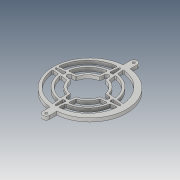
# Autodesk Inventor part: verticalThrusterCover2
Saved by Autodesk Inventor 2018 (Build 220112000, 112)
## iProperties
Created: 2020-02-09
Part Number: verticalThrusterCover2
Material: Generic
Document SubType Name: Modeling
Designer: anirudh
Density: 1 g/cm^3
Appearance: Default
Author: anirudh
Autodesk Inventor part; units mm, degrees
ref_plane "YZ Plane" through (0, 0, 0) normal (1, 0, 0) x (0, 1, 0)
ref_plane "XZ Plane" through (0, 0, 0) normal (0, 1, 0) x (-1, 0, 0)
ref_plane "XY Plane" through (0, 0, 0) normal (0, 0, 1) x (1, 0, 0)
sketch "Sketch1" plane through (0, 0, 0) normal (0, 1, 0) x (-1, 0, 0)
  circle A0 centre (0, -63.5) radius 1.75
  circle A1 centre (0, 63.5) radius 1.75
  circle A2 centre (0, -63.5) radius 1.75
  circle A3 centre (0, 63.5) radius 1.75
  arc A4 (5.08, 63.5) -> (-5.08, 63.5) centre (0, 63.5) ccw
  arc A5 (-5.08, -63.5) -> (5.08, -63.5) centre (0, -63.5) ccw
  line L0 (5.08, 63.5) -> (5.08, 53.0975)
  line L1 (5.08, -53.0975) -> (5.08, -63.5)
  line L2 (-5.08, -63.5) -> (-5.08, -53.0975)
  line L3 (-5.08, 53.0975) -> (-5.08, 63.5)
  arc A6 (-5.08, 53.0975) -> (-5.08, -53.0975) centre (0, 0) ccw
  arc A7 (5.08, -53.0975) -> (5.08, 53.0975) centre (0, 0) ccw
  arc A8 (-0.1848, -27.646) -> (6.1284, -27.646) centre (2.9718, -27.305) ccw
  line L4 (6.8199, -21.2443) -> (6.1284, -27.646)
  line L5 (-0.1848, -27.646) -> (-0.8763, -21.2443)
  line L6 (30.6178, -3.1566) -> (24.2161, -3.8481)
  line L7 (24.2161, 3.8481) -> (30.6178, 3.1566)
  arc A9 (30.6178, -3.1566) -> (30.6178, 3.1566) centre (30.2768, 0) ccw
  line L8 (6.1284, 27.646) -> (6.8199, 21.2443)
  line L9 (-0.8763, 21.2443) -> (-0.1848, 27.646)
  arc A10 (6.1284, 27.646) -> (-0.1848, 27.646) centre (2.9718, 27.305) ccw
  line L10 (-24.6742, 3.1566) -> (-18.2725, 3.8481)
  line L11 (-18.2725, -3.8481) -> (-24.6742, -3.1566)
  arc A11 (-24.6742, 3.1566) -> (-24.6742, -3.1566) centre (-24.3332, 0) ccw
  arc A12 (24.2161, 3.8481) -> (6.8199, 21.2443) centre (2.9718, 0) ccw
  arc A13 (-0.8763, 21.2443) -> (-18.2725, 3.8481) centre (2.9718, 0) ccw
  arc A14 (-18.2725, -3.8481) -> (-0.8763, -21.2443) centre (2.9718, 0) ccw
  arc A15 (6.8199, -21.2443) -> (24.2161, -3.8481) centre (2.9718, 0) ccw
  dimension "d34" = 360
  constraints: 24 end point, 24 point on circle, 16 centre point, 4 coincident, 4 vertical, 2 concentric, 33 other
extrude "Extrusion2" add sketch "Sketch1" along normal blind 5.08
sketch "Sketch2" plane through (0, 5.08, 0) normal (0, 1, 0) x (1, 0, 0)
  arc A0 (-26.7955, -6.763) -> (-9.7348, -23.8237) centre (-2.9718, 0) ccw
  arc A1 (-37.2778, -5.6307) -> (-8.6025, -34.306) centre (-2.9718, 0) ccw
  arc A2 (-40.5429, -5.278) -> (-8.2498, -37.5711) centre (-2.9718, 0) ccw
  line L0 (-9.7348, -23.8237) -> (-8.6025, -34.306)
  line L1 (-8.2498, -37.5711) -> (-7.2268, -47.0423)
  line L2 (-26.7955, -6.763) -> (-37.2778, -5.6307)
  line L3 (-40.5429, -5.278) -> (-50.0141, -4.255)
  arc A3 (-50.0141, -4.255) -> (-7.2268, -47.0423) centre (-2.9718, 0) ccw
  arc A4 (-49.0619, 1.1643) -> (-49.0619, -1.1643) centre (-48.9362, 0) ccw
  line L4 (-36.0852, -2.5661) -> (-49.0619, -1.1643)
  line L5 (-36.0852, 2.5661) -> (-49.0619, 1.1643)
  arc A5 (-36.0852, 2.5661) -> (-36.0852, -2.5661) centre (-30.2768, 0) ccw
  line L6 (34.5993, -5.278) -> (44.0705, -4.255)
  line L7 (20.8519, -6.763) -> (31.3342, -5.6307)
  arc A6 (1.2832, -47.0423) -> (44.0705, -4.255) centre (-2.9718, 0) ccw
  arc A7 (2.3062, -37.5711) -> (34.5993, -5.278) centre (-2.9718, 0) ccw
  arc A8 (2.6589, -34.306) -> (31.3342, -5.6307) centre (-2.9718, 0) ccw
  arc A9 (3.7912, -23.8237) -> (20.8519, -6.763) centre (-2.9718, 0) ccw
  line L8 (3.7912, -23.8237) -> (2.6589, -34.306)
  line L9 (2.3062, -37.5711) -> (1.2832, -47.0423)
  line L10 (-0.4057, -33.1134) -> (-1.8075, -46.0901)
  arc A10 (-5.5379, -33.1134) -> (-0.4057, -33.1134) centre (-2.9718, -27.305) ccw
  line L11 (-5.5379, -33.1134) -> (-4.1361, -46.0901)
  arc A11 (-4.1361, -46.0901) -> (-1.8075, -46.0901) centre (-2.9718, -45.9644) ccw
  line L12 (2.3062, 37.5711) -> (1.2832, 47.0423)
  line L13 (3.7912, 23.8237) -> (2.6589, 34.306)
  arc A12 (44.0705, 4.255) -> (1.2832, 47.0423) centre (-2.9718, 0) ccw
  arc A13 (34.5993, 5.278) -> (2.3062, 37.5711) centre (-2.9718, 0) ccw
  arc A14 (31.3342, 5.6307) -> (2.6589, 34.306) centre (-2.9718, 0) ccw
  arc A15 (20.8519, 6.763) -> (3.7912, 23.8237) centre (-2.9718, 0) ccw
  line L14 (20.8519, 6.763) -> (31.3342, 5.6307)
  line L15 (34.5993, 5.278) -> (44.0705, 4.255)
  line L16 (30.1416, 2.5661) -> (43.1183, 1.1643)
  arc A16 (30.1416, -2.5661) -> (30.1416, 2.5661) centre (24.3332, 0) ccw
  line L17 (30.1416, -2.5661) -> (43.1183, -1.1643)
  arc A17 (43.1183, -1.1643) -> (43.1183, 1.1643) centre (42.9926, 0) ccw
  line L18 (-40.5429, 5.278) -> (-50.0141, 4.255)
  line L19 (-26.7955, 6.763) -> (-37.2778, 5.6307)
  arc A18 (-7.2268, 47.0423) -> (-50.0141, 4.255) centre (-2.9718, 0) ccw
  arc A19 (-8.2498, 37.5711) -> (-40.5429, 5.278) centre (-2.9718, 0) ccw
  arc A20 (-8.6025, 34.306) -> (-37.2778, 5.6307) centre (-2.9718, 0) ccw
  arc A21 (-9.7348, 23.8237) -> (-26.7955, 6.763) centre (-2.9718, 0) ccw
  line L20 (-9.7348, 23.8237) -> (-8.6025, 34.306)
  line L21 (-8.2498, 37.5711) -> (-7.2268, 47.0423)
  line L22 (-5.5379, 33.1134) -> (-4.1361, 46.0901)
  arc A22 (-0.4057, 33.1134) -> (-5.5379, 33.1134) centre (-2.9718, 27.305) ccw
  line L23 (-0.4057, 33.1134) -> (-1.8075, 46.0901)
  arc A23 (-1.8075, 46.0901) -> (-4.1361, 46.0901) centre (-2.9718, 45.9644) ccw
  point P0 (0, 0)
  point P1 (-6.8199, -21.2443)
  point P2 (-6.1284, -27.646)
  point P3 (-24.2161, -3.8481)
  point P4 (-30.6178, 3.1566)
  point P5 (-24.2161, 3.8481)
  dimension "d49" = 360
  constraints: 48 end point, 48 point on circle, 24 centre point, 10 coincident, 1 tangent, 121 other
extrude "Extrusion3" cut sketch "Sketch2" against normal blind 5.08
fillet "Fillet3" radius 1.27 46 edges at (-7.2268, 2.54, 47.0423) (-8.2498, 2.54, 37.5711) (-8.6025, 2.54, 34.306) (-9.7348, 2.54, 23.8237) (-0.4057, 2.54, 33.1134) (-5.5379, 2.54, 33.1134) (-26.7955, 2.54, 6.763) (-37.2778, 2.54, 5.6307) (-40.5429, 2.54, 5.278) (-50.0141, 2.54, 4.255) (-36.0852, 2.54, 2.5661) (-36.0852, 2.54, -2.5661) (-50.0141, 2.54, -4.255) (-40.5429, 2.54, -5.278) (-37.2778, 2.54, -5.6307) (-26.7955, 2.54, -6.763) (-24.2161, 2.54, 3.8481) (-24.2161, 2.54, -3.8481) (0.8763, 2.54, 21.2443) (-6.8199, 2.54, 21.2443) (2.6589, 2.54, 34.306) (3.7912, 2.54, 23.8237) (2.3062, 2.54, 37.5711) (1.2832, 2.54, 47.0423) (44.0705, 2.54, 4.255) (34.5993, 2.54, 5.278) (31.3342, 2.54, 5.6307) (20.8519, 2.54, 6.763) (18.2725, 2.54, 3.8481) (18.2725, 2.54, -3.8481) (0.8763, 2.54, -21.2443) (20.8519, 2.54, -6.763) (31.3342, 2.54, -5.6307) (44.0705, 2.54, -4.255) (3.7912, 2.54, -23.8237) (2.6589, 2.54, -34.306) (2.3062, 2.54, -37.5711) (1.2832, 2.54, -47.0423) (-0.4057, 2.54, -33.1134) (-5.5379, 2.54, -33.1134) (-7.2268, 2.54, -47.0423) (-8.2498, 2.54, -37.5711) (-8.6025, 2.54, -34.306) (-9.7348, 2.54, -23.8237) (30.1416, 2.54, 2.5661) (30.1416, 2.54, -2.5661)
body "Solid2"
